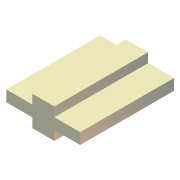
# Autodesk Inventor part: Lift Slider
Saved by Autodesk Inventor 2011 (Build 150239000, 239)
## iProperties
Created: 2014-09-14
Part Number: Lift Slider
Document SubType Name: Modeling
Designer: Family Room
Density: 1 g/cm^3
Author: Family Room
Autodesk Inventor part; units mm, degrees
ref_plane "YZ Plane" through (0, 0, 0) normal (1, 0, 0) x (0, 1, 0)
ref_plane "XZ Plane" through (0, 0, 0) normal (0, 1, 0) x (-1, 0, 0)
ref_plane "XY Plane" through (0, 0, 0) normal (0, 0, 1) x (1, 0, 0)
sketch "Sketch1" plane through (0, 0, 0) normal (0, 0, 1) x (1, 0, 0)
  line L0 (0, 0) -> (20, 0)
  line L1 (20, 0) -> (20, 3)
  line L2 (20, 3) -> (0, 3)
  line L3 (0, 3) -> (0, 0)
  line L4 (7, 3) -> (13, 3)
  line L5 (13, 3) -> (13, 5.54)
  line L6 (13, 5.54) -> (7, 5.54)
  line L7 (7, 5.54) -> (7, 3)
  line L8 (7, 0) -> (13, 0)
  line L9 (13, 0) -> (13, -2.54)
  line L10 (13, -2.54) -> (7, -2.54)
  line L11 (7, -2.54) -> (7, 0)
  dimension "d0" = 20
  dimension "d1" = 3
  dimension "d2" = 6
  dimension "d3" = 2.54
  dimension "d4" = 6
  dimension "d5" = 2.54
  dimension "d6" = 7
  dimension "d7" = 7
  constraints: 24 end point, 6 parallel, 3 horizontal, 3 perpendicular, 2 point on line
  measures "d0" distance of L2.end L1.end
  measures "d1" distance of L1.end L0.end
  measures "d2" distance of L6.end L5.end
  measures "d3" distance of L5.end L4.end
  measures "d4" distance of L9.end L10.end
  measures "d5" distance of L8.end L9.end
  measures "d6" distance between parallel lines of L3 L7
  measures "d7" distance between parallel lines of L3 L11
extrude "Extrusion1" add sketch "Sketch1" along normal blind 25.4
ref_plane "Work Plane1" through (10, 3, 0) normal (1, 0, 0) x (0, 0, -1)
body "Solid1"
